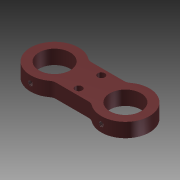
# Autodesk Inventor part: 13_0204_047
Saved by Autodesk Inventor 2012 SP1 (Build 160190100, 190)
## iProperties
Created: 2013-04-10
Part Number: 13_0204_047
Material: Default
Document SubType Name: Modeling
Designer: vogel
Density: 1 g/cm^3
Author: vogel
Autodesk Inventor part; units mm, degrees
ref_plane "YZ Plane" through (0, 0, 0) normal (1, 0, 0) x (0, 1, 0)
ref_plane "XY Plane" through (0, 0, 0) normal (0, 0, 1) x (1, 0, 0)
sketch "Skizze1" plane through (0, 0, 0) normal (0, 0, 1) x (1, 0, 0)
  line L0 (-58.8, 0) -> (58.8, 0) projected
  line L1 (0, -24.5) -> (0, 24.5) projected
  circle A0 centre (-25, 0) radius 11
  circle A1 centre (25, 0) radius 11
  arc A2 (-14.6978, 13.5227) -> (-14.6978, -13.5227) centre (-25, 0) ccw
  arc A3 (14.6978, -13.5227) -> (14.6978, 13.5227) centre (25, 0) ccw
  line L2 (11.6677, -12.5) -> (-11.6677, -12.5)
  line L3 (-11.6677, 12.5) -> (11.6677, 12.5)
  arc A4 (-11.6677, -12.5) -> (-14.6978, -13.5227) centre (-11.6677, -17.5) ccw
  arc A5 (14.6978, -13.5227) -> (11.6677, -12.5) centre (11.6677, -17.5) ccw
  arc A6 (11.6677, 12.5) -> (14.6978, 13.5227) centre (11.6677, 17.5) ccw
  arc A7 (-14.6978, 13.5227) -> (-11.6677, 12.5) centre (-11.6677, 17.5) ccw
  point P0 (0, 0)
  point P1 (-13.4783, -12.5)
  point P2 (13.4783, 12.5)
  point P3 (13.4783, -12.5)
  point P4 (-13.4783, 12.5)
  dimension "d0" = 50
  dimension "d1" = 22
  dimension "d2" = 34
  dimension "d4" = 25
  dimension "d5" = 5
  dimension "d6" = 6
  constraints: 16 point on circle, 8 centre point, 8 tangent, 6 point on line, 5 equal radius, 4 end point, 2 coincident, 1 horizontal, 1 parallel, 2 other
  measures "d0" distance of A1.centre A0.centre
  measures "d1" diameter of A0
  measures "d2" diameter of A2
  measures "d4" distance between parallel lines of L2 L3
  measures "d5" radius of A4
  measures "d6" radial gap between concentric circles of A2 A0
extrude "Extrusion1" add sketch "Skizze1" along normal blind 10 contours A2 A7 L3 L1 L0 A0 | L0 A0 L1 L2 A4 A2 | L1 L3 A6 A3 L0 A1 | L0 A1 A3 A5 L2 L1
ref_plane "Arbeitsebene1" through (25, -17, 0) normal (0, 1, 0) x (-1, 0, 0)
sketch "Skizze2" plane through (25, -17, 0) normal (0, 1, 0) x (-1, 0, 0)
  line L0 (-33.8, 0) -> (83.8, 0) projected
  line L1 (25, -2) -> (25, 12) projected
  line L2 (39.6978, 10) -> (67, 10) projected
  line L3 (-17, 10) -> (10.3022, 10) projected
  line L4 (-17, 0) -> (-17, 10) projected
  line L5 (67, 0) -> (67, 10) projected
  line L6 (67, 5) -> (-17, 5)
  point P0 (25, 0)
  point P1 (50, 5)
  point P2 (0, 5)
  dimension "d9" = 50
  constraints: 2 end point, 2 midpoint, 2 point on line, 1 symmetric about line
  measures "d9" distance of point (0, 5) point (50, 5)
hole "Bohrung1" at (-25, -17, 5) at (25, -17, 5) direction (0, 1, 0) diameter 3.242 depth 8 tip angle 118 thread size "M4x0.7" class "6H" standard "ISO Metric profile"
sketch "Skizze3" plane through (0, 0, 10) normal (0, 0, 1) x (1, 0, 0)
  circle A0 centre (0, -8) radius 1.5 projected
  circle A1 centre (0, 8) radius 1.5 projected
  point P0 (0, 0)
  constraints: 2 coincident
hole "Bohrung2" at (0, 8, 10) at (0, -8, 10) direction (0, 0, -1) diameter 5 end through all
